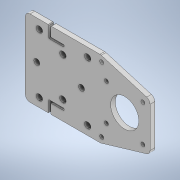
# Autodesk Inventor part: podstawa_prawa
Saved by Autodesk Inventor 2020 (Build 240168000, 168)
## iProperties
Created: 2020-09-29
Part Number: podstawa_prawa
Material: Ogólny
Document SubType Name: Konstrukcja blachowa
Designer: szymo
Density: 1 g/cm^3
Sheet Metal Rule: Domyślny_mm
Appearance: Domyślna
Author: szymo
Autodesk Inventor part; units mm, degrees
ref_plane "YZ Plane" through (0, 0, 0) normal (1, 0, 0) x (0, 1, 0)
ref_plane "XZ Plane" through (0, 0, 0) normal (0, 1, 0) x (-1, 0, 0)
ref_plane "XY Plane" through (0, 0, 0) normal (0, 0, 1) x (1, 0, 0)
sketch "Szkic1" plane through (0, 0, 0) normal (0, 0, 1) x (1, 0, 0)
  line L0 (0, 61) -> (0, 4)
  line L1 (106, 15.4829) -> (106, 49.5171)
  line L2 (103.141, 53.3509) -> (64.5584, 64.8338)
  line L3 (103.141, 11.6491) -> (64.5584, 0.1662)
  arc A0 (4, 65) -> (0, 61) centre (4, 61) ccw
  arc A1 (64.5584, 64.8338) -> (63.4174, 65) centre (63.4174, 61) ccw
  arc A2 (106, 49.5171) -> (103.141, 53.3509) centre (102, 49.5171) ccw
  arc A3 (103.141, 11.6491) -> (106, 15.4829) centre (102, 15.4829) ccw
  arc A4 (63.4174, 0) -> (64.5584, 0.1662) centre (63.4174, 4) ccw
  arc A5 (0, 4) -> (4, 0) centre (4, 4) ccw
  line L4 (0, 0) -> (20, 0)
  line L5 (20, 0.5) -> (20, 9.5)
  line L6 (20.5, 10) -> (32.5, 10)
  line L7 (33, 9.5) -> (33, 8.75)
  line L8 (32.5, 8.25) -> (22.25, 8.25)
  line L9 (21.75, 7.75) -> (21.75, 0.5)
  line L10 (4, 0) -> (19.5, 0)
  line L11 (22.25, 0) -> (63.4174, 0)
  arc A6 (19.5, 0) -> (20, 0.5) centre (19.5, 0.5) ccw
  arc A7 (20.5, 10) -> (20, 9.5) centre (20.5, 9.5) ccw
  arc A8 (33, 9.5) -> (32.5, 10) centre (32.5, 9.5) ccw
  arc A9 (32.5, 8.25) -> (33, 8.75) centre (32.5, 8.75) ccw
  arc A10 (22.25, 8.25) -> (21.75, 7.75) centre (22.25, 7.75) ccw
  arc A11 (21.75, 0.5) -> (22.25, 0) centre (22.25, 0.5) ccw
  line L12 (20, 64.5) -> (20, 55.5)
  line L13 (20.5, 55) -> (32.5, 55)
  line L14 (33, 55.5) -> (33, 56.25)
  line L15 (32.5, 56.75) -> (22.25, 56.75)
  line L16 (21.75, 57.25) -> (21.75, 64.5)
  arc A12 (20, 64.5) -> (19.5, 65) centre (19.5, 64.5) ccw
  arc A13 (20, 55.5) -> (20.5, 55) centre (20.5, 55.5) ccw
  arc A14 (32.5, 55) -> (33, 55.5) centre (32.5, 55.5) ccw
  arc A15 (33, 56.25) -> (32.5, 56.75) centre (32.5, 56.25) ccw
  arc A16 (21.75, 57.25) -> (22.25, 56.75) centre (22.25, 57.25) ccw
  arc A17 (22.25, 65) -> (21.75, 64.5) centre (22.25, 64.5) ccw
  line L17 (63.4174, 65) -> (22.25, 65)
  line L18 (19.5, 65) -> (4, 65)
  circle A18 centre (65, 5) radius 1.7
  circle A19 centre (65, 60) radius 1.7
  circle A20 centre (69, 48) radius 1.7
  circle A21 centre (100, 48) radius 1.7
  circle A22 centre (69, 17) radius 1.7
  circle A23 centre (100, 17) radius 1.7
  circle A24 centre (84.5, 32.5) radius 12
  circle A25 centre (9.85, 32.5) radius 2.5
  circle A26 centre (47.85, 32.5) radius 2.5
  arc A27 (11.75, 60) -> (11.75, 55) centre (11.75, 57.5) ccw
  arc A28 (12.25, 55) -> (12.25, 60) centre (12.25, 57.5) ccw
  line L19 (11.75, 60) -> (12.25, 60)
  line L20 (11.75, 55) -> (12.25, 55)
  arc A29 (52.75, 60) -> (52.75, 55) centre (52.75, 57.5) ccw
  arc A30 (53.25, 55) -> (53.25, 60) centre (53.25, 57.5) ccw
  line L21 (52.75, 60) -> (53.25, 60)
  line L22 (52.75, 55) -> (53.25, 55)
  arc A31 (11.75, 10) -> (11.75, 5) centre (11.75, 7.5) ccw
  arc A32 (12.25, 5) -> (12.25, 10) centre (12.25, 7.5) ccw
  line L23 (11.75, 5) -> (12.25, 5)
  line L24 (11.75, 10) -> (12.25, 10)
  arc A33 (52.75, 10) -> (52.75, 5) centre (52.75, 7.5) ccw
  arc A34 (53.25, 5) -> (53.25, 10) centre (53.25, 7.5) ccw
  line L25 (52.75, 5) -> (53.25, 5)
  line L26 (52.75, 10) -> (53.25, 10)
  arc A35 (31.75, 51.5) -> (31.75, 46.5) centre (31.75, 49) ccw
  arc A36 (32.25, 46.5) -> (32.25, 51.5) centre (32.25, 49) ccw
  line L27 (31.75, 51.5) -> (32.25, 51.5)
  line L28 (31.75, 46.5) -> (32.25, 46.5)
  arc A37 (31.75, 18.5) -> (31.75, 13.5) centre (31.75, 16) ccw
  arc A38 (32.25, 13.5) -> (32.25, 18.5) centre (32.25, 16) ccw
  line L29 (31.75, 13.5) -> (32.25, 13.5)
  line L30 (31.75, 18.5) -> (32.25, 18.5)
  point P0 (106, 12.5)
  point P1 (106, 52.5)
  point P2 (20, 10)
  point P3 (33, 10)
  point P4 (33, 8.25)
  point P5 (21.75, 8.25)
  point P6 (21.75, 56.75)
  dimension "d2" = 106
  dimension "d3" = 40
  dimension "d5" = 4
  dimension "d6" = 20
  dimension "d7" = 10
  dimension "d8" = 13
  dimension "d9" = 1.75
  dimension "d10" = 11.25
  dimension "d11" = 0.5
  dimension "d12" = 3.4
  dimension "d13" = 65
  dimension "d14" = 5
  dimension "d16" = 3.4
  dimension "d18" = 69
  dimension "d19" = 3.4
  dimension "d20" = 3.4
  dimension "d21" = 3.4
  dimension "d24" = 69
  dimension "d25" = 31
  dimension "d26" = 31
  dimension "d27" = 24
  dimension "d28" = 84.5
  dimension "d29" = 5
  dimension "d30" = 5
  dimension "d31" = 9.85
  dimension "d32" = 38
  dimension "d33" = 5
  dimension "d35" = 5
  dimension "d36" = 9.25
  dimension "d37" = 5
  dimension "d39" = 5
  dimension "d40" = 35.5
  dimension "d42" = 5
  dimension "d47" = 5
  dimension "d48" = 5
  measures "d2" distance between parallel lines of L0 L1
  measures "d3" distance of point (106, 12.5) point (106, 52.5)
  measures "d5" radius of A0
  measures "d6" distance of L4.start L4.end
  measures "d7" distance of L4.end point (20, 10)
  measures "d8" distance of point (20, 10) point (33, 10)
  measures "d9" distance of point (33, 10) point (33, 8.25)
  measures "d10" distance of point (33, 8.25) point (21.75, 8.25)
  measures "d11" radius of A6
  measures "d12" diameter of A18
  measures "d13" distance from line of L0 A18.centre
  measures "d14" distance from line of L11 A18.centre
  measures "d16" diameter of A20
  measures "d18" distance from line of L0 A20.centre
  measures "d19" diameter of A21
  measures "d20" diameter of A22
  measures "d21" diameter of A23
  measures "d24" distance from line of L0 A22.centre
  measures "d25" distance of A22.centre A23.centre
  measures "d26" distance of A20.centre A21.centre
  measures "d27" diameter of A24
  measures "d28" distance from line of L0 A24.centre
  measures "d29" diameter of A25
  measures "d30" diameter of A26
  measures "d31" distance from line of L0 A25.centre
  measures "d32" distance of A26.centre A25.centre
  measures "d33" diameter of A27
  measures "d35" diameter of A28
  measures "d36" distance edge to line of A27 L0
  measures "d37" distance from line of L19.end L18
  measures "d39" diameter of A29
  measures "d42" diameter of A30
  measures "d47" diameter of A35
  measures "d48" diameter of A36
extrude "Płyta1" add sketch "Szkic1" along normal blind 4
equation "\"d49\" = Grubość"
equation "\"PromieńGięcia\" = Grubość"
equation "\"SzerokośćGięciaPodcięcia\" = Grubość"
equation "\"GłębokośćGięciaPodcięcia\" = 0.5 * Grubość"
equation "\"RozmiarPodcięciaNarożnika\" = 4 * Grubość"
equation "\"MinimalnaPozostałość\" = 2 * Grubość"
equation "\"PromieńPrzejścia\" = PromieńGięcia"
equation "\"Rozmiar_promienia_Jacobiego\" = PromieńGięcia"
equation "\"Wielk_odstępu\" = Grubość"
equation "\"Grubość\" = 4"
